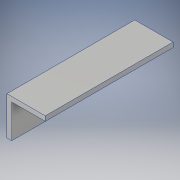
# Autodesk Inventor part: bepf_platforma_wspornik_poziomy
Saved by Autodesk Inventor 2017 (Build 210142000, 142)
## iProperties
Created: 2016-11-24
Part Number: bepf_platforma_wspornik_poziomy
Material: Aluminium 6061
Document SubType Name: Modeling
Designer: gagato
Density: 2.7 g/cm^3
Appearance: Aluminium — płaski
Mass: 3.60603 g
Surface Area: 19.8475 cm^2
Volume: 1.33557 cm^3
Author: gagato
Autodesk Inventor part; units mm, degrees
ref_plane "YZ Plane" through (0, 0, 0) normal (1, 0, 0) x (0, 1, 0)
ref_plane "XZ Plane" through (0, 0, 0) normal (0, 1, 0) x (-1, 0, 0)
ref_plane "XY Plane" through (0, 0, 0) normal (0, 0, 1) x (1, 0, 0)
sketch "Szkic1" plane through (0, 0, 0) normal (0, 0, 1) x (1, 0, 0)
  line L0 (0, 0) -> (0, -12)
  line L1 (0, -12) -> (1.5, -12)
  line L2 (1.5, -12) -> (1.5, -1.5)
  line L3 (1.5, -1.5) -> (12, -1.5)
  line L4 (12, -1.5) -> (12, 0)
  line L5 (12, 0) -> (0, 0)
  dimension "d0" = 12
  dimension "d1" = 1.5
  dimension "d2" = 10.5
  dimension "d3" = 10.5
  constraints: 12 end point, 3 perpendicular, 1 horizontal, 1 parallel, 1 vertical
  measures "d0" distance of L0.start L0.end
  measures "d1" distance of L0.end L1.end
  measures "d2" distance of L1.end L2.end
  measures "d3" distance of L2.end L3.end
extrude "Wyciągnięcie proste1" add sketch "Szkic1" along normal mid plane 40
sketch "Szkic2" plane through (1.5, -12, 20) normal (1, 0, 0) x (0, 0, -1)
  line L0 (40, 0) -> (0, 0) projected
  line L1 (40, 0) -> (0, 0) construction
  line L2 (20, 0) -> (20, 5) construction
  point P0 (20, 12)
  dimension "d6" = 5
  constraints: 2 end point, 1 coincident, 1 midpoint, 1 vertical
  measures "d6" distance of L2.start L2.end
hole "Otwór1" at (1.5, -7, 0) direction (-1, 0, 0) diameter 3.5 end through all
